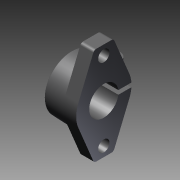
# Autodesk Inventor part: SHF18b
Saved by Autodesk Inventor 2011 SP1 (Build 150282100, 282)
## iProperties
Created: 2016-11-23
Part Number: SHF18b
Catalog Web Link: www.cadenas.de
Description: SHFT, SHFM, SHFSS, SHF, SHFD-b-Shaft Supports - Flanged Type (Precision Casting) - Standard Type
Vendor: MISUMI
Document SubType Name: Modeling
Designer: psAdmin
Manufacturer: MISUMI
Mass: 16.072 g
Surface Area: 67.7011 cm^2
Volume: 16.072 cm^3
Density: 1 g/cm^3
Category: PARTsolutions
Company: MISUMI
Title: SHF18b
Author: Cadenas PARTsolutions
Comments: Shaft Supports - Flanged Type (Precision Casting) - Standard Type
PSOL_IDENT_0: {$CADENAS_DATA\23d-libs\misumi\metric\02_shaft_supports\shft.prj},185 {VTYP=3D},{NB=SHF18b},{LINA=SH
PSOL_IDENT_1: F18b},{NN=SHFT, SHFM, SHFSS, SHF, SHFD-b},{DATE=17.06.2016 05:45:11},{GEOMDATE=30.07.2008 06:54:00},
PSOL_IDENT_2: {VERSION=},{LINEID=110},{LINESUBID=-1},{WBVAR=MAT,ST}  {NB=SHF18b},{LINA=SHF18b},{KT=DUMMY},{PN=SHF1
PSOL_IDENT_3: 8},{TYPE=SHF},{MAT=514},{ST=Clear Anodize},{AC=Hexagon Socket Head Cap Screws (1 Pc.) ( Stainless St
PSOL_IDENT_4: eel) },{D=18},{L=60},{T=20},{TT=8},{H=37},{A=34},{L1=48},{DD=7.0},{DD1=10},{D1=24},{TT1=2.0},{B=22},
PSOL_IDENT_5: {C=2.5},{BB1=28},{BB2=5},{BB3=14},{HH=15.0},{M=M5},{THMD=5},{THDMIN=4.134},{ST0='Clear Anodize','Cle
PSOL_IDENT_6: ar Anodize'},{MASS=38},{MAT1='514','Aluminum Casting Alloy 514.0'},{DM=5},{HM=20.000},{MASSS=110},{M
PSOL_IDENT_7: ASSA=38}
NN: SHFT, SHFM, SHFSS, SHF, SHFD-b
NT: Shaft Supports - Flanged Type (Precision Casting) - Standard Type
NB: SHF18b
NBSYN: $PN.b
LINA: SHF18b
PN: SHF18
MAT: Aluminum Casting Alloy 514.0
ST: Clear Anodize
AC: Hexagon Socket Head Cap Screws (1 Pc.) ( Stainless Steel)
D: 18
L: 60
T: 20
TT: 8
H: 37
A: 34
L1: 48
DD: 7.0
DD1: 10
D1: 24
TT1: 2.0
B: 22
C: 2.5
HH: 15.0
M: M5
MASS: 38
SUPPLIER: MISUMI
ARTICLENO: SHF18b
BOMINFO: SHF18b
CREATOR: CADENAS GmbH
Autodesk Inventor part; units mm, degrees
sketch "Sketch_1" plane through (0, 0, 0) normal (1, 0, 0) x (0, 1, 0)
  line L0 (4.6379, 30) -> (-4.6379, 30)
  arc A0 (-4.6379, 30) -> (-6.4857, 28.7654) centre (-4.6379, 28) ccw
  line L1 (-6.4857, 28.7654) -> (-15.706, 6.5056)
  arc A1 (-15.706, 6.5056) -> (-17, 0) centre (0, 0) ccw
  arc A2 (-17, 0) -> (-15.706, -6.5056) centre (0, 0) ccw
  line L2 (-15.706, -6.5056) -> (-6.4857, -28.7654)
  arc A3 (-6.4857, -28.7654) -> (-4.6379, -30) centre (-4.6379, -28) ccw
  line L3 (-4.6379, -30) -> (4.6379, -30)
  arc A4 (4.6379, -30) -> (6.4857, -28.7654) centre (4.6379, -28) ccw
  line L4 (6.4857, -28.7654) -> (15.706, -6.5056)
  arc A5 (15.706, -6.5056) -> (17, 0) centre (0, 0) ccw
  arc A6 (17, 0) -> (15.706, 6.5056) centre (0, 0) ccw
  line L5 (15.706, 6.5056) -> (6.4857, 28.7654)
  arc A7 (6.4857, 28.7654) -> (4.6379, 30) centre (4.6379, 28) ccw
  constraints: 16 point on circle, 12 end point, 8 centre point
extrude "Extrusion1" add sketch "Sketch_1" against normal blind 8
sketch "Sketch_2" plane through (0, 0, 0) normal (0, 0, 1) x (1, 0, 0)
  line L0 (-8, 0) -> (-20, 0)
  line L1 (-20, 0) -> (-20, 16.0904)
  arc A0 (-19.5097, 16.5981) -> (-20, 16.0904) centre (-19.492, 16.0904) ccw
  line L2 (-19.5097, 16.5981) -> (-8, 17)
  line L3 (-8, 17) -> (-8, 0)
  line L4 (-8, 0) -> (-20, 0)
  constraints: 10 end point, 2 point on circle, 1 centre point
revolve "Revolution1" add sketch "Sketch_2" angle 360 about axis through (-8, 0, 0) along (1, 0, 0)
sketch "Sketch_3" plane through (0, 0, 0) normal (0, 0, 1) x (1, 0, 0)
  circle A0 centre (-10, 15) radius 5
  constraints: 1 centre point
extrude "Extrusion2" add sketch "Sketch_3" along normal mid plane 22
sketch "Sketch_4" plane through (0, 0, 11) normal (0, 0, 1) x (1, 0, 0)
  line L0 (-20, 10) -> (-10, 10)
  arc A0 (-10, 10) -> (-15, 15) centre (-10, 15) ccw
  line L1 (-15, 15) -> (-20, 15)
  line L2 (-20, 15) -> (-20, 10)
  constraints: 6 end point, 2 point on circle, 1 centre point
extrude "Extrusion3" cut sketch "Sketch_4" along normal blind 11
sketch "Sketch_5" plane through (0, 0, 0) normal (1, 0, 0) x (0, 1, 0)
  line L0 (0, 1.25) -> (0, -1.25)
  line L1 (0, -1.25) -> (37, -1.25)
  line L2 (37, -1.25) -> (37, 1.25)
  line L3 (37, 1.25) -> (0, 1.25)
  constraints: 8 end point
extrude "Extrusion4" cut sketch "Sketch_5" against normal blind 20
sketch "Sketch_6" plane through (0, 0, 0) normal (0, 0, 1) x (1, 0, 0)
  line L0 (0, 0) -> (-20, 0)
  line L1 (-20, 0) -> (-20, 12)
  line L2 (-20, 12) -> (-18, 12)
  line L3 (-18, 12) -> (-18, 9)
  line L4 (-18, 9) -> (0, 9)
  line L5 (0, 9) -> (0, 0)
  line L6 (0, 0) -> (-20, 0)
  constraints: 14 end point
revolve "Revolution2" cut sketch "Sketch_6" angle 360 about axis through (0, 0, 0) along (1, 0, 0)
sketch "Sketch_7" plane through (-10, 0, 0) normal (1, 0, 0) x (0, 0, -1)
  line L0 (16.5, 15) -> (1.25, 15)
  line L1 (1.25, 15) -> (1.25, 17.5)
  line L2 (1.25, 17.5) -> (1.683, 17.067)
  line L3 (1.683, 17.067) -> (10.567, 17.067)
  line L4 (10.567, 17.067) -> (11.1, 17.6)
  line L5 (11.1, 17.6) -> (16.5, 17.6)
  line L6 (16.5, 17.6) -> (16.5, 15)
  line L7 (16.5, 15) -> (1.25, 15)
  constraints: 16 end point
revolve "Revolution3" cut sketch "Sketch_7" angle 360 about axis through (-10, 15, -16.5) along (0, 0, -1)
thread "Thread1" size "M5x0.8" class "6H" standard "ISO Metric profile" full length
sketch "Sketch_8" plane through (-10, 0, 0) normal (1, 0, 0) x (0, 0, -1)
  line L0 (-1.25, 15) -> (-11, 15)
  line L1 (-11, 15) -> (-11, 17.5)
  line L2 (-11, 17.5) -> (-10.567, 17.067)
  line L3 (-10.567, 17.067) -> (-1.683, 17.067)
  line L4 (-1.683, 17.067) -> (-1.25, 17.5)
  line L5 (-1.25, 17.5) -> (-1.25, 15)
  line L6 (-1.25, 15) -> (-11, 15)
  constraints: 14 end point
revolve "Revolution4" cut sketch "Sketch_8" angle 360 about axis through (-10, 15, 1.25) along (0, 0, -1)
thread "Thread2" size "M5x0.8" class "6H" standard "ISO Metric profile" full length
sketch "Sketch9" plane through (0, 0, 0) normal (1, 0, 0) x (0, 0, -1)
  point P0 (24, 0)
hole "Hole1" at (0, 0, -24) direction (-1, 0, 0) diameter 7 depth 8
sketch "Sketch10" plane through (0, 0, 0) normal (1, 0, 0) x (0, 0, -1)
  point P0 (-24, 0)
hole "Hole2" at (0, 0, 24) direction (-1, 0, 0) diameter 7 depth 8
ref_plane "body_screw_XY" through (-10, 15, 11) normal (0, 0, 1) x (1, 0, 0)
ref_plane "body_screw_YZ" through (-10, 15, 11) normal (1, 0, 0) x (0, 1, 0)
ref_plane "body_screw_ZX" through (-10, 15, 11) normal (0, 1, 0) x (0, 0, 1)
body "Solid1"
